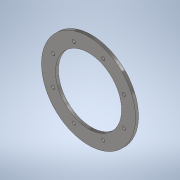
# Autodesk Inventor part: Придав перегородки1
Saved by Autodesk Inventor 2021 (Build 250183000, 183)
## iProperties
Created: 2020-11-17
Part Number: Придав перегородки1
Material: Сталь, высокопрочная, низколегированная
Document SubType Name: Modeling
Designer: Тимоха
Density: 7.85 g/cm^3
Appearance: Сталь — полированная
Mass: 3121.1 g
Surface Area: 996.56 cm^2
Volume: 397.592 cm^3
Author: Тимоха
Autodesk Inventor part; units mm, degrees
ref_plane "YZ Plane" through (0, 0, 0) normal (1, 0, 0) x (0, 1, 0)
ref_plane "XZ Plane" through (0, 0, 0) normal (0, 1, 0) x (-1, 0, 0)
ref_plane "XY Plane" through (0, 0, 0) normal (0, 0, 1) x (1, 0, 0)
sketch "Эскиз1" plane through (0, 0, 0) normal (0, 0, 1) x (1, 0, 0)
  circle A0 centre (0, 0) radius 112.5
  circle A1 centre (0, 0) radius 160
  dimension "d0" = 225
  dimension "d1" = 320
  constraints: 2 centre point, 2 coincident
  measures "d0" diameter of A0
  measures "d1" diameter of A1
extrude "Выдавливание1" add sketch "Эскиз1" along normal blind 10
sketch "Эскиз2" plane through (0, 0, 10) normal (0, 0, 1) x (1, 0, 0)
  line L0 (0, 0) -> (120.1043, 49.7488)
  line L1 (-224, 0) -> (224, 0) projected
  dimension "d4" = 130
  dimension "d5" = 22.5
  constraints: 2 end point
  measures "d4" distance of L0.start L0.end
  measures "d5" angle of L1 L0
hole "Отверстие1" at (120.1043, 49.7488, 10) direction (0, 0, -1) diameter 12 end through all
pattern_circular "Круговой массив1" count 8 over 360 about axis through (0, 0, 0) along (0, 0, 1) of "Отверстие1"
